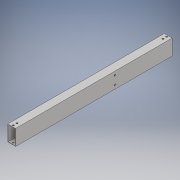
# Autodesk Inventor part: nhk48
Saved by Autodesk Inventor 2019 (Build 230136000, 136)
## iProperties
Created: 2022-02-28
Part Number: nhk48
Material: 一般
Document SubType Name: Sheet Metal
Designer: yuta
Density: 1 g/cm^3
Sheet Metal Rule: Default_mm
Appearance: 既定
Author: yuta
Autodesk Inventor part; units mm, degrees
ref_plane "YZ Plane" through (0, 0, 0) normal (1, 0, 0) x (0, 1, 0)
ref_plane "XZ Plane" through (0, 0, 0) normal (0, 1, 0) x (-1, 0, 0)
ref_plane "XY Plane" through (0, 0, 0) normal (0, 0, 1) x (1, 0, 0)
sketch "スケッチ1" plane through (0, 0, 0) normal (0, 0, 1) x (1, 0, 0)
  line L0 (0, 0) -> (15, 0)
  line L1 (15, 0) -> (15, 30)
  line L2 (15, 30) -> (0, 30)
  line L3 (0, 30) -> (0, 0)
  line L4 (1, 1) -> (14, 1)
  line L5 (14, 1) -> (14, 29)
  line L6 (14, 29) -> (1, 29)
  line L7 (1, 29) -> (1, 1)
  dimension "d0" = 15
  dimension "d1" = 30
  dimension "d2" = 13
  dimension "d3" = 28
  dimension "d4" = 1
  dimension "d5" = 1
  constraints: 16 end point, 4 parallel, 2 horizontal, 2 perpendicular
  measures "d0" distance of L2.end L1.end
  measures "d1" distance of L1.end L0.end
  measures "d2" distance of L6.end L5.end
  measures "d3" distance of L5.end L4.end
  measures "d4" distance between parallel lines of L3 L7
  measures "d5" distance between parallel lines of L0 L4
extrude "押し出し1" add sketch "スケッチ1" along normal blind 300
sketch "スケッチ2" plane through (0, 30, 0) normal (0, 1, 0) x (1, 0, 0)
  circle A0 centre (7.5, -3) radius 1.6
  line L0 (15, 0) -> (15, -300) projected
  line L1 (15, 0) -> (0, 0) projected
  circle A1 centre (7.5, -10) radius 1.6
  line L2 (0, -150) -> (15, -150) construction
  line L3 (15, -300) -> (0, -300) projected
  circle A2 centre (7.5, -297) radius 1.6
  circle A3 centre (7.5, -290) radius 1.6
  dimension "d8" = 3.2
  dimension "d9" = 7.5
  dimension "d10" = 3
  dimension "d11" = 3.2
  dimension "d12" = 7
  dimension "d13" = 7.5
  dimension "d14" = 150
  constraints: 4 centre point, 2 end point, 2 symmetric about line, 1 midpoint, 1 perpendicular, 2 other
  measures "d8" diameter of A0
  measures "d9" distance from line of L0 A0.centre
  measures "d10" distance from line of L1 A0.centre
  measures "d11" diameter of A1
  measures "d12" distance of A0.centre A1.centre
  measures "d13" distance from line of L0 A1.centre
  measures "d14" distance between parallel lines of L3 L2
hole "穴1" at (7.5, 30, 297) at (7.5, 30, 290) at (7.5, 30, 10) at (7.5, 30, 3) direction (0, -1, 0) diameter 3.2 depth 30
sketch "スケッチ3" plane through (15, 0, 0) normal (1, 0, 0) x (0, 0, -1)
  circle A0 centre (-109.5, 23) radius 1.6
  line L0 (0, 0) -> (0, 30) projected
  line L1 (0, 30) -> (-300, 30) projected
  circle A1 centre (-109.5, 7) radius 1.6
  line L2 (0, 0) -> (-300, 0) projected
  dimension "d22" = 3.2
  dimension "d23" = 109.5
  dimension "d24" = 7
  dimension "d25" = 3.2
  dimension "d26" = 16
  dimension "d27" = 7
  constraints: 2 centre point
  measures "d22" diameter of A0
  measures "d23" distance from line of L0 A0.centre
  measures "d24" distance from line of L1 A0.centre
  measures "d25" diameter of A1
  measures "d26" distance of A1.centre A0.centre
  measures "d27" distance from line of L2 A1.centre
hole "穴2" at (15, 23, 109.5) at (15, 7, 109.5) direction (-1, 0, 0) diameter 3.2 depth 15
equation "\"BendRadius\" = Thickness"
equation "\"BendReliefWidth\" = Thickness"
equation "\"BendReliefDepth\" = 0.5 * Thickness"
equation "\"CornerReliefSize\" = 4 * Thickness"
equation "\"MinimumRemnant\" = 2 * Thickness"
equation "\"TransitionRadius\" = BendRadius"
equation "\"JacobiRadiusSize\" = BendRadius"
equation "\"GapSize\" = Thickness"
equation "\"Thickness\" = 0.5"
